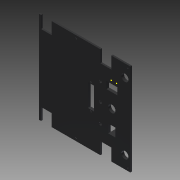
# Autodesk Inventor part: vrchna_platna
Saved by Autodesk Inventor 2015 (Build 190159000, 159)
## iProperties
Created: 2015-06-09
Part Number: vrchna_platna
Material: ABS Plastic
Document SubType Name: Modeling
Designer: Jufo
Density: 1 g/cm^3
Appearance: Smooth - White
Author: Jufo
Autodesk Inventor part; units mm, degrees
ref_plane "YZ Plane" through (0, 0, 0) normal (1, 0, 0) x (0, 1, 0)
ref_plane "XZ Plane" through (0, 0, 0) normal (0, 1, 0) x (-1, 0, 0)
ref_plane "XY Plane" through (0, 0, 0) normal (0, 0, 1) x (1, 0, 0)
sketch "Sketch1" plane through (0, 0, 0) normal (0, 1, 0) x (-1, 0, 0)
  line L0 (-34.9372, 39.6819) -> (0.5628, 39.6819)
  line L1 (0.5628, 39.6819) -> (0.5628, 17.1819)
  line L2 (0.5628, 17.1819) -> (20.5628, 17.1819)
  line L3 (20.5628, 17.1819) -> (20.5628, 39.6819)
  line L4 (20.5628, 39.6819) -> (110.5628, 39.6819)
  line L5 (110.5628, 39.6819) -> (110.5628, 17.1819)
  line L6 (110.5628, 17.1819) -> (130.5628, 17.1819)
  line L7 (130.5628, 17.1819) -> (130.5628, 39.6819)
  line L8 (130.5628, 39.6819) -> (134.5628, 39.6819)
  line L9 (134.5628, 39.6819) -> (134.5628, -130.3181)
  line L10 (-34.9372, 39.6819) -> (-34.9372, -130.3181)
  line L11 (-34.9372, -130.3181) -> (0.5628, -130.3181)
  line L12 (0.5628, -130.3181) -> (0.5628, -107.8181)
  line L13 (0.5628, -107.8181) -> (20.5628, -107.8181)
  line L14 (20.5628, -107.8181) -> (20.5628, -130.3181)
  line L15 (20.5628, -130.3181) -> (110.5628, -130.3181)
  line L16 (110.5628, -130.3181) -> (110.5628, -107.8181)
  line L17 (110.5628, -107.8181) -> (130.5628, -107.8181)
  line L18 (130.5628, -107.8181) -> (130.5628, -130.3181)
  line L19 (130.5628, -130.3181) -> (134.5628, -130.3181)
  point P0 (0, 0)
  dimension "d0" = 35.5
  dimension "d2" = 22.5
  dimension "d3" = 22.5
  dimension "d4" = 22.5
  dimension "d5" = 22.5
  dimension "d6" = 170
  dimension "d7" = 170
  dimension "d8" = 20
  dimension "d9" = 20
  dimension "d10" = 4
  dimension "d32" = 90
  dimension "d33" = 90
  dimension "d34" = 4
  dimension "d42" = 22.5
  dimension "d43" = 22.5
  dimension "d44" = 22.5
  constraints: 40 end point, 7 parallel, 2 collinear, 1 horizontal, 1 perpendicular
  measures "d0" distance of L0.start L0.end
  measures "d2" distance of L0.end L1.end
  measures "d3" distance of L2.end L3.end
  measures "d4" distance of L4.end L5.end
  measures "d5" distance of L6.end L7.end
  measures "d6" distance of L0.start L10.end
  measures "d7" distance of L8.end L9.end
  measures "d8" distance of L1.end L2.end
  measures "d9" distance of L5.end L6.end
  measures "d10" distance of L7.end L8.end
  measures "d32" distance of L3.end L4.end
  measures "d33" distance of L14.end L15.end
  measures "d34" distance of L18.end L9.end
  measures "d42" distance of L13.end L14.end
  measures "d43" distance of L11.end L12.end
  measures "d44" distance of L15.end L16.end
extrude "Extrusion1" add sketch "Sketch1" along normal blind 3
sketch "Sketch2" plane through (0, 3, 0) normal (0, 1, 0) x (1, 0, 0)
  line L0 (-0.5628, -39.6819) -> (34.9372, -39.6819) projected
  line L1 (34.9372, -39.6819) -> (34.9372, 130.3181) projected
  line L2 (34.9372, 130.3181) -> (-0.5628, 130.3181) projected
  line L3 (-0.5628, 130.3181) -> (-0.5628, 107.8181) projected
  line L4 (-0.5628, 107.8181) -> (-20.5628, 107.8181) projected
  line L5 (-20.5628, 107.8181) -> (-20.5628, 130.3181) projected
  line L6 (-20.5628, 130.3181) -> (-110.5628, 130.3181) projected
  line L7 (-110.5628, 130.3181) -> (-110.5628, 107.8181) projected
  line L8 (-110.5628, 107.8181) -> (-130.5628, 107.8181) projected
  line L9 (-130.5628, 107.8181) -> (-130.5628, 130.3181) projected
  line L10 (-130.5628, 130.3181) -> (-134.5628, 130.3181) projected
  line L11 (-134.5628, 130.3181) -> (-134.5628, -39.6819) projected
  line L12 (-134.5628, -39.6819) -> (-130.5628, -39.6819) projected
  line L13 (-130.5628, -39.6819) -> (-130.5628, -17.1819) projected
  line L14 (-130.5628, -17.1819) -> (-110.5628, -17.1819) projected
  line L15 (-110.5628, -17.1819) -> (-110.5628, -39.6819) projected
  line L16 (-110.5628, -39.6819) -> (-20.5628, -39.6819) projected
  line L17 (-20.5628, -39.6819) -> (-20.5628, -17.1819) projected
  line L18 (-20.5628, -17.1819) -> (-0.5628, -17.1819) projected
  line L19 (-0.5628, -17.1819) -> (-0.5628, -39.6819) projected
  line L20 (32.4372, 127.8181) -> (32.4372, -37.1819)
  line L21 (32.4372, -37.1819) -> (3.9372, -37.1819)
  line L22 (3.9372, -37.1819) -> (3.9372, -10.6819)
  line L23 (3.9372, -10.6819) -> (-25.0628, -10.6819)
  line L24 (-25.0628, -10.6819) -> (-25.0628, -37.1819)
  line L25 (-25.0628, -37.1819) -> (-106.0628, -37.1819)
  line L26 (-106.0628, -37.1819) -> (-106.0628, -10.6819)
  line L27 (-106.0628, -10.6819) -> (-134.5628, -10.6819)
  line L28 (34.9372, 45.3181) -> (-27.5518, 45.3181)
  line L29 (32.4372, 127.8181) -> (3.9372, 127.8181)
  line L30 (3.9372, 127.8181) -> (3.9372, 101.3181)
  line L31 (3.9372, 101.3181) -> (-25.0628, 101.3181)
  line L32 (-25.0628, 101.3181) -> (-25.0628, 127.8181)
  line L33 (-25.0628, 127.8181) -> (-106.0628, 127.8181)
  line L34 (-106.0628, 127.8181) -> (-106.0628, 101.3181)
  line L35 (-106.0628, 101.3181) -> (-134.5628, 101.3181)
  line L36 (-134.5628, 101.3181) -> (-134.5628, 130.3181)
  line L37 (-134.5628, -10.6819) -> (-134.5628, -39.6819)
  point P0 (0, 0)
  dimension "d13" = 6.5
  dimension "d14" = 4.5
  dimension "d15" = 2.5
  dimension "d17" = 4.5
  dimension "d18" = 6.5
  dimension "d19" = 4.5
  dimension "d20" = 2.5
  dimension "d21" = 2.5
  dimension "d112" = 6.5
  dimension "d113" = 6.5
  dimension "d114" = 4.5
  dimension "d115" = 4
  dimension "d116" = 4.5
  dimension "d117" = 4.5
  constraints: 36 end point, 7 symmetric about line, 5 parallel, 4 perpendicular, 2 collinear, 1 midpoint, 1 point on line
  measures "d13" distance between parallel lines of L14 L27
  measures "d14" distance between parallel lines of L15 L26
  measures "d15" distance between parallel lines of L16 L25
  measures "d17" distance between parallel lines of L17 L24
  measures "d18" distance between parallel lines of L18 L23
  measures "d19" distance between parallel lines of L19 L22
  measures "d20" distance between parallel lines of L0 L21
  measures "d21" distance between parallel lines of L1 L20
  measures "d112" distance between parallel lines of L4 L31
  measures "d113" distance between parallel lines of L8 L35
  measures "d114" distance between parallel lines of L7 L34
  measures "d115" distance between parallel lines of L9 L11
  measures "d116" distance between parallel lines of L5 L32
  measures "d117" distance between parallel lines of L3 L30
extrude "Extrusion2" add sketch "Sketch2" along normal blind 2 contours L20 L21 L22 L23 L24 L25 L26 L27 L11 L35 L34 L33 L32 L31 L30 L29
sketch "Sketch3" plane through (0, 5, 0) normal (0, 1, 0) x (1, 0, 0)
  line L0 (-106.0628, -37.1819) -> (-25.0628, -37.1819) projected
  line L1 (3.9372, -37.1819) -> (32.4372, -37.1819) projected
  line L2 (32.4372, -37.1819) -> (32.4372, 127.8181) projected
  line L3 (32.4372, -37.1819) -> (32.4372, -31.6819)
  line L4 (32.4372, -31.6819) -> (26.9372, -31.6819)
  line L5 (26.9372, -31.6819) -> (26.9372, -37.1819)
  line L6 (26.9372, -31.6819) -> (26.9372, -34.6819)
  line L7 (26.9372, -34.6819) -> (29.9372, -34.6819)
  circle A0 centre (29.9372, -34.6819) radius 1.5
  line L8 (32.4372, 45.3181) -> (-36.6937, 45.3181)
  line L9 (-65.5628, -37.1819) -> (-62.5628, -37.1819)
  line L10 (-62.5628, -37.1819) -> (-62.5628, -31.6819)
  line L11 (-62.5628, -31.6819) -> (-68.0628, -31.6819)
  line L12 (-68.0628, -31.6819) -> (-68.0628, -37.1819)
  line L13 (-65.3128, -31.6819) -> (-65.3128, -34.6819)
  circle A1 centre (-65.3128, -34.6819) radius 1.5
  circle A2 centre (29.9372, 125.3181) radius 1.5
  circle A3 centre (-65.3128, 125.3181) radius 1.5
  point P0 (0, 0)
  dimension "d26" = 5.5
  dimension "d27" = 5.5
  dimension "d28" = 3
  dimension "d29" = 3
  dimension "d30" = 3
  dimension "d36" = 3
  dimension "d37" = 5.5
  dimension "d38" = 3
  dimension "d39" = 3
  dimension "d48" = 5.5
  constraints: 22 end point, 5 perpendicular, 5 point on line, 4 centre point, 3 midpoint, 3 parallel, 2 coincident, 2 symmetric about line, 2 other
  measures "d26" distance of L1.end L3.end
  measures "d27" distance of L3.end L4.end
  measures "d28" distance of L4.end L6.end
  measures "d29" distance of L6.end L7.end
  measures "d30" diameter of A0
  measures "d36" distance of L9.start L9.end
  measures "d37" distance of L10.end L11.end
  measures "d38" distance of L13.start L13.end
  measures "d39" diameter of A1
  measures "d48" distance of L11.end L12.end
extrude "Extrusion3" cut sketch "Sketch3" against normal blind 5 contours A0 | A1 | A2 | A3
sketch "Sketch5" plane through (0, 0, 0) normal (0, -1, 0) x (1, 0, 0)
  point P0 (0, 0)
sketch "Sketch6" plane through (0, 0, 0) normal (0, -1, 0) x (1, 0, 0)
  line L0 (3.9372, 37.1819) -> (32.4372, 37.1819) projected
  line L1 (22.9372, 22.6819) -> (22.9372, -113.3181)
  line L2 (3.9372, -127.8181) -> (32.4372, -127.8181) projected
  line L3 (32.4372, -127.8181) -> (32.4372, 37.1819) projected
  circle A0 centre (22.9372, -113.3181) radius 6.75
  circle A1 centre (22.9372, 22.6819) radius 6.75
  line L4 (34.9372, 39.6819) -> (34.9372, -130.3181) projected
  point P0 (0, 0)
  dimension "d49" = 136
  dimension "d52" = 165
  dimension "d54" = 14.5
  dimension "d55" = 13.5
  dimension "d56" = 13.5
  dimension "d118" = 14.5
  dimension "d120" = 12
  dimension "d121" = 12
  constraints: 2 centre point, 2 coincident, 2 end point
  measures "d49" distance of L1.start L1.end
  measures "d52" distance between parallel lines of L0 L2
  measures "d54" distance from line of L2 L1.end
  measures "d55" diameter of A0
  measures "d56" diameter of A1
  measures "d118" distance from line of L0 A1.centre
  measures "d120" distance from line of L4 A0.centre
  measures "d121" distance from line of L4 A1.centre
extrude "Extrusion4" cut sketch "Sketch6" against normal blind 5
sketch "Sketch7" plane through (0, 5, 0) normal (0, 1, 0) x (1, 0, 0)
  line L0 (32.4372, -37.1819) -> (32.4372, 127.8181) projected
  line L1 (32.4372, 45.3181) -> (7.4372, 45.3181)
  circle A0 centre (0.6872, 45.3181) radius 6.75
  point P0 (0, 0)
  dimension "d59" = 25
  dimension "d61" = 13.5
  constraints: 2 end point, 1 centre point, 1 horizontal, 1 midpoint
  measures "d59" distance of L1.start L1.end
  measures "d61" diameter of A0
extrude "Extrusion5" cut sketch "Sketch7" against normal blind 5
sketch "Sketch8" plane through (0, 5, 0) normal (0, 1, 0) x (1, 0, 0)
  point P0 (0, 0)
sketch "Sketch9" plane through (0, 5, 0) normal (0, 1, 0) x (1, 0, 0)
  line L0 (7.4372, 52.0681) -> (7.4372, 32.0681)
  line L1 (7.4372, 32.0681) -> (9.4372, 32.0681)
  line L2 (9.4372, 32.0681) -> (9.4372, 52.0681)
  line L3 (9.4372, 52.0681) -> (7.4372, 52.0681)
  point P0 (0, 0)
  dimension "d64" = 20
  dimension "d65" = 2
  constraints: 8 end point, 3 perpendicular, 1 vertical
  measures "d64" distance of L0.start L0.end
  measures "d65" distance of L0.end L1.end
extrude "Extrusion6" add sketch "Sketch9" along normal blind 10
sketch "Sketch10" plane through (9.4372, 5, -32.0681) normal (1, 0, 0) x (0, 0, -1)
  point P0 (-32.0681, -5)
sketch "Sketch11" plane through (7.4372, 5, -45.3181) normal (-1, 0, 0) x (0, 0, 1)
  line L0 (13.25, 0) -> (0, 0) projected
  line L1 (6.625, 0) -> (6.625, 10)
  line L2 (-6.75, 10) -> (13.25, 10) projected
  circle A0 centre (10.25, 6) radius 1
  line L3 (13.25, 0) -> (13.25, 10) projected
  point P0 (45.3181, -5)
  dimension "d68" = 2
  dimension "d69" = 6
  dimension "d70" = 3
  constraints: 2 end point, 1 centre point, 1 midpoint, 1 point on line, 1 vertical
  measures "d68" diameter of A0
  measures "d69" distance from line of L0 A0.centre
  measures "d70" distance from line of A0.centre L3
extrude "Extrusion7" cut sketch "Sketch11" against normal blind 2 contours A0
sketch "Sketch12" plane through (0, 0, 0) normal (0, -1, 0) x (1, 0, 0)
  circle A0 centre (0.6872, -45.3181) radius 6.75 projected
  line L0 (0.4581, -72.0642) -> (-6.3419, -72.0642)
  line L1 (-6.3419, -72.0642) -> (-6.3419, -88.0642)
  line L2 (-6.3419, -88.0642) -> (7.2581, -88.0642)
  line L3 (7.2581, -88.0642) -> (7.2581, -72.0642)
  line L4 (7.2581, -72.0642) -> (0.4581, -72.0642)
  point P0 (0, 0)
  dimension "d74" = 6.8
  dimension "d75" = 16
  dimension "d76" = 13.6
  constraints: 10 end point, 4 perpendicular, 1 horizontal, 1 point on line
  measures "d74" distance of L0.start L0.end
  measures "d75" distance of L0.end L1.end
  measures "d76" distance of L1.end L2.end
extrude "Extrusion8" cut sketch "Sketch12" against normal blind 5 contours L4 L3 L2 L1 L0
sketch "Sketch13" plane through (0, 0, 0) normal (0, -1, 0) x (1, 0, 0)
  circle A0 centre (0.6872, -45.3181) radius 6.75 projected
  line L0 (0.6872, -38.5681) -> (0.6872, -18.5681)
  line L1 (0.6872, -18.5681) -> (-9.3128, -18.5681)
  line L2 (-9.3128, -18.5681) -> (-9.3128, -5.5681)
  line L3 (-9.3128, -5.5681) -> (10.6872, -5.5681)
  line L4 (10.6872, -5.5681) -> (10.6872, -18.5681)
  line L5 (10.6872, -18.5681) -> (0.6872, -18.5681)
  point P0 (0, 0)
  point P1 (7.4372, -45.3181)
  dimension "d79" = 20
  dimension "d80" = 10
  dimension "d81" = 13
  dimension "d82" = 20
  constraints: 12 end point, 5 perpendicular, 1 point on circle, 1 point on line, 1 vertical
  measures "d79" distance of L0.start L0.end
  measures "d80" distance of L0.end L1.end
  measures "d81" distance of L1.end L2.end
  measures "d82" distance of L2.end L3.end
extrude "Extrusion9" cut sketch "Sketch13" against normal blind 5 contours L1 L2 L3 L4 L5
sketch "Sketch14" plane through (0, 5, 0) normal (0, 1, 0) x (1, 0, 0)
  line L0 (7.2581, 72.0642) -> (7.2581, 70.0642)
  line L1 (7.2581, 70.0642) -> (-6.3419, 70.0642)
  line L2 (-6.3419, 70.0642) -> (-6.3419, 72.0642)
  line L3 (7.2581, 88.0642) -> (7.2581, 90.0642)
  line L4 (7.2581, 90.0642) -> (-6.3419, 90.0642)
  line L5 (-6.3419, 90.0642) -> (-6.3419, 88.0642)
  line L6 (7.2581, 72.0642) -> (-6.3419, 72.0642)
  line L7 (-6.3419, 88.0642) -> (-6.3419, 72.0642) projected
  line L8 (7.2581, 88.0642) -> (-6.3419, 88.0642)
  point P0 (0, 0)
  dimension "d85" = 2
  dimension "d86" = 2
  constraints: 16 end point, 5 perpendicular, 2 vertical, 1 horizontal
  measures "d85" distance of L0.start L0.end
  measures "d86" distance of L3.start L3.end
extrude "Extrusion10" add sketch "Sketch14" along normal blind 15
sketch "Sketch15" plane through (0, 0, 0) normal (0, -1, 0) x (1, 0, 0)
  line L0 (-9.3128, -18.5681) -> (-9.3128, -5.5681) projected
  circle A0 centre (-20.5628, -80.0642) radius 2.5
  circle A1 centre (-20.5628, -45.3181) radius 2.5
  circle A2 centre (-20.5628, -12.0681) radius 2.5
  point P0 (0, 0)
  dimension "d90" = 5
  dimension "d91" = 5
  dimension "d92" = 5
  constraints: 3 centre point
  measures "d90" diameter of A0
  measures "d91" diameter of A1
  measures "d92" diameter of A2
extrude "Extrusion11" cut sketch "Sketch15" against normal blind 5
sketch "Sketch16" plane through (0, 0, 0) normal (0, -1, 0) x (1, 0, 0)
  line L0 (-43.7628, -66.0681) -> (-32.5628, -66.0681)
  line L1 (-32.5628, -66.0681) -> (-32.5628, -24.5681)
  line L2 (-32.5628, -24.5681) -> (-43.7628, -24.5681)
  line L3 (-43.7628, -24.5681) -> (-43.7628, -66.0681)
  line L4 (32.4372, -127.8181) -> (32.4372, 37.1819) projected
  line L5 (-20.5628, 39.6819) -> (-110.5628, 39.6819) projected
  line L6 (-110.5628, -130.3181) -> (-20.5628, -130.3181) projected
  circle A0 centre (-38.2628, -21.5681) radius 1.5
  circle A1 centre (-38.2628, -69.0681) radius 1.5
  point P0 (0, 0)
  point P1 (-17.9642, -27.5954)
  point P2 (-17.9642, 1.6449)
  point P3 (-17.9642, 1.6449)
  point P4 (-17.9642, -27.5954)
  dimension "d97" = 41.5
  dimension "d98" = 11.2
  dimension "d99" = 65
  dimension "d100" = 64.25
  dimension "d101" = 64.25
  dimension "d102" = 3
  dimension "d103" = 3
  dimension "d104" = 3
  dimension "d105" = 3
  dimension "d106" = 5.5
  dimension "d107" = 5.5
  dimension "d108" = 5.7
  dimension "d109" = 5.7
  constraints: 8 end point, 2 centre point, 2 coincident, 2 parallel, 1 horizontal, 1 perpendicular, 4 other
  measures "d97" distance of L2.end L0.start
  measures "d98" distance of L1.end L2.end
  measures "d99" distance between parallel lines of L4 L1
  measures "d100" distance between parallel lines of L5 L2
  measures "d101" distance between parallel lines of L6 L0
  measures "d102" diameter of A0
  measures "d103" diameter of A1
  measures "d104" distance from line of L2 A0.centre
  measures "d105" distance from line of L0 A1.centre
  measures "d106" distance from line of L3 A0.centre
  measures "d107" distance from line of L3 A1.centre
  measures "d108" distance from line of L1 A0.centre
  measures "d109" distance from line of L1 A1.centre
extrude "Extrusion12" cut sketch "Sketch16" against normal blind 10
equation "\"d3\" = d2"
equation "\"d4\" = d2"
equation "\"d5\" = d2"
equation "\"d42\" = d2"
equation "\"d43\" = d2"
equation "\"d44\" = d2"
equation "\"d17\" = d14"
equation "\"d19\" = d14"
equation "\"d20\" = d15"
equation "\"d21\" = d20"
body "Solid1"
